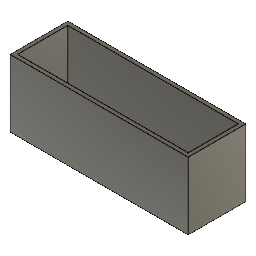
nerf based hopper housing bottom v6 (Autodesk Fusion 360 design; units mm, degrees)
Autodesk Fusion 360 part; units mm, degrees
box "BoxPrimitive1" add length 76.2 width 234.95 height 88.9 placed x (0, -1, 0) y (1, 0, 0) z (0, 0, 1) at (0, 0, 0)
shell "Shell1" thickness 5.08 removed faces 1 at (78.3167, -25.4, 88.9)
sketch "flywheel axle" plane through (5.08, 0, 0) normal (1, 0, 0) x (0, 1, 0)
  line L0 (-5.08, 5.08) -> (-5.08, 88.9)
  line L1 (-5.08, 88.9) -> (-71.12, 88.9)
  line L2 (-71.12, 88.9) -> (-71.12, 5.08)
  line L3 (-71.12, 5.08) -> (-5.08, 5.08)
  line L4 (-38.1, 88.9) -> (-38.1, 5.08) construction
  line L5 (-71.12, 46.99) -> (-5.08, 46.99) construction
  circle A0 centre (-38.1, 46.99) radius 3.1
  point P0 (-38.1, 46.99)
  dimension "d10" = 6.2
  constraint midpoint L1 L4.start
  constraint midpoint L3 L4.end
  constraint midpoint L2 L5.start
  constraint midpoint L0 L5.end
  constraint midpoint L4 P0
  constraint coincident P0 A0.centre
  measures "d10" diameter of A0
extrude "Extrude1" add sketch "flywheel axle" along normal blind 228.6 contours A0
sketch "tube slot" plane through (0, 0, 0) normal (0, 1, 0) x (-1, 0, 0)
  line L0 (-234.95, 88.9) -> (-234.95, 0)
  line L1 (-234.95, 0) -> (0, 0)
  line L2 (0, 0) -> (0, 88.9)
  line L3 (0, 88.9) -> (-234.95, 88.9)
  line L4 (-233.68, 11.3178) -> (-1.905, 11.3178)
  line L5 (-1.905, 11.3178) -> (-1.905, 5.08)
  line L6 (-1.905, 5.08) -> (-233.68, 5.08)
  line L7 (-233.68, 5.08) -> (-233.68, 11.3178)
  dimension "d11" = 231.775
  dimension "d13" = 6.2378
  dimension "d14" = 1.27
  dimension "d15" = 5.08
  constraint horizontal L4
  constraint vertical L5
  constraint horizontal L6
  constraint vertical L7
  measures "d11" distance of L4.start L4.end
  measures "d13" distance of L4.end L5.end
  measures "d14" distance of L0 L7
  measures "d15" distance of L1 L6
extrude "Extrude2" cut sketch "tube slot" against normal blind 12.7 contours L4 L5 L6 L7
named bodies: "bottom hopper"
